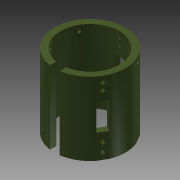
# Autodesk Inventor part: 知能ロボコン外筒改1.2
Saved by Autodesk Inventor 2013 (Build 170138000, 138)
## iProperties
Created: 2014-05-28
Part Number: 知能ロボコン外筒改1.2
Material: ABS プラスチック
Document SubType Name: Modeling
Designer: horumo136
Density: 1 g/cm^3
Author: horumo136
Autodesk Inventor part; units mm, degrees
sketch "スケッチ1" plane through (0, 0, 0) normal (0, 0, 1) x (1, 0, 0)
  circle A0 centre (0, 0) radius 13
  line L0 (0, 13) -> (0, 33)
  circle A1 centre (0, 0) radius 33
  circle A2 centre (0, 0) radius 40
  dimension "d0" = 26
  dimension "d2" = 20
  dimension "d3" = 80
  constraints: 3 coincident, 2 end point, 2 vertical alignment, 1 centre point, 1 vertical, 4 other
  measures "d2" distance of L0.start L0.end
  measures "d3" diameter of A2
extrude "押し出し1" add sketch "スケッチ1" along normal blind 145 contours A2
sketch "スケッチ2" plane through (0, 0, 0) normal (0, 0, -1) x (-1, 0, 0)
  circle A0 centre (0, 0) radius 33 projected
  circle A1 centre (0, 0) radius 40 projected
  line L0 (5.4, 32.5552) -> (-5.4, 32.5552)
  line L1 (0, 0) -> (-10.5703, 0)
  arc A2 (5.4, 32.5552) -> (-5.4, 32.5552) centre (0, 0) ccw
  line L2 (-5.4, 32.5552) -> (5.4, 32.5552)
  line L3 (5.4, 32.5552) -> (5.4, 32.5552)
  line L4 (5.4, 32.5552) -> (-5.4, 32.5552)
  line L5 (-5.4, 32.5552) -> (-5.4, 32.5552)
  line L6 (-5.4, 32.5552) -> (5.4, 32.5552)
  line L7 (5.4, 32.5552) -> (5.4, 33)
  line L8 (5.4, 33) -> (-5.4, 33)
  line L9 (-5.4, 33) -> (-5.4, 32.5552)
  line L10 (-30.8936, -11.6011) -> (-25.4936, -20.9541)
  line L11 (-30.8936, -11.6011) -> (-31.2788, -11.8235)
  line L12 (-31.2788, -11.8235) -> (-25.8788, -21.1765)
  line L13 (-25.8788, -21.1765) -> (-25.4936, -20.9541)
  line L14 (25.4936, -20.9541) -> (30.8936, -11.6011)
  line L15 (25.4936, -20.9541) -> (25.8788, -21.1765)
  line L16 (25.8788, -21.1765) -> (31.2788, -11.8235)
  line L17 (31.2788, -11.8235) -> (30.8936, -11.6011)
  line L18 (-30.8936, -11.6011) -> (-31.2788, -11.8235)
  line L19 (-31.2788, -11.8235) -> (-25.8788, -21.1765)
  line L20 (-25.8788, -21.1765) -> (-25.4936, -20.9541)
  line L21 (-25.4936, -20.9541) -> (-30.8936, -11.6011)
  line L22 (25.4936, -20.9541) -> (25.8788, -21.1765)
  line L23 (25.8788, -21.1765) -> (31.2788, -11.8235)
  line L24 (31.2788, -11.8235) -> (30.8936, -11.6011)
  line L25 (30.8936, -11.6011) -> (25.4936, -20.9541)
  dimension "d6" = 10.8
  dimension "d8" = 10.8
  dimension "d13" = 360
  constraints: 52 end point, 8 parallel, 6 perpendicular, 5 point on circle, 3 horizontal, 1 centre point, 1 collinear, 1 concentric, 31 other
  measures "d6" distance of L0.start L0.end
  measures "d8" distance of L4.end L3.end
extrude "押し出し2" cut sketch "スケッチ2" against normal blind 145 contours L0 A0 | A0 L8 L7 | L17 L16 A0 | A0 L14 | A0 L9 L8 | L16 L15 A0 | L10 A0 | A0 L12 L11 | L13 L12 A0
sketch "スケッチ3" plane through (-5.4, 33, 0) normal (0, -1, 0) x (1, 0, 0)
  line L0 (10.8, 0) -> (10.8, 145) projected
  line L1 (5.4, 0) -> (5.4, 19.5)
  line L2 (5.4, 19.5) -> (5.4, 24.2)
  line L3 (5.4, 24.2) -> (5.4, 74.8)
  circle A0 centre (5.4, 24.2) radius 1.5
  circle A1 centre (5.4, 74.8) radius 1.5
  line L4 (5.4, 74.8) -> (5.4, 79.9)
  line L5 (5.4, 79.9) -> (5.4, 84.6)
  circle A2 centre (5.4, 84.6) radius 1.5
  line L6 (5.4, 84.6) -> (5.4, 135.2)
  circle A3 centre (5.4, 135.2) radius 1.5
  dimension "d15" = 19.5
  dimension "d16" = 4.7
  dimension "d17" = 50.6
  dimension "d18" = 3
  dimension "d19" = 3
  dimension "d20" = 5.1
  dimension "d21" = 4.7
  dimension "d22" = 3
  dimension "d23" = 50.6
  dimension "d24" = 3
  constraints: 12 end point, 5 collinear, 4 centre point, 4 coincident, 1 parallel
  measures "d15" distance of L1.start L1.end
  measures "d16" distance of L1.end L2.end
  measures "d17" distance of L2.end L3.end
  measures "d18" diameter of A0
  measures "d19" diameter of A1
  measures "d20" distance of L4.start L4.end
  measures "d21" distance of L4.end L5.end
  measures "d22" diameter of A2
  measures "d23" distance of L6.start L6.end
  measures "d24" diameter of A3
hole "穴1" at (0, 33, 24.2) at (0, 33, 74.8) at (0, 33, 84.6) at (0, 33, 135.2) direction (0, 1, 0) diameter 3 depth 8 tip angle 118
pattern_circular "円形状パターン1" count 3 over 360 about axis through (0, 0, 0) along (0, 0, 1) of "穴1"
sketch "スケッチ4" plane through (0, 0, 0) normal (0, 0, -1) x (-1, 0, 0)
  circle A0 centre (0, 0) radius 40 projected
  line L0 (30.8936, -11.6011) -> (31.2788, -11.8235) projected
  line L1 (31.2788, -11.8235) -> (25.8788, -21.1765) projected
  line L2 (25.8788, -21.1765) -> (25.4936, -20.9541) projected
  arc A1 (-25.4936, -20.9541) -> (25.4936, -20.9541) centre (0, 0) ccw projected
  line L3 (-25.4936, -20.9541) -> (-25.8788, -21.1765) projected
  line L4 (-25.8788, -21.1765) -> (-31.2788, -11.8235) projected
  line L5 (-31.2788, -11.8235) -> (-30.8936, -11.6011) projected
  arc A2 (-5.4, 32.5552) -> (-30.8936, -11.6011) centre (0, 0) ccw projected
  line L6 (-5.4, 32.5552) -> (-5.4, 33) projected
  line L7 (-5.4, 33) -> (5.4, 33) projected
  line L8 (5.4, 33) -> (5.4, 32.5552) projected
  arc A3 (30.8936, -11.6011) -> (5.4, 32.5552) centre (0, 0) ccw projected
  point P0 (0, 40)
  point P1 (-34.641, 20)
  point P2 (-34.641, -20)
  point P3 (0, -40)
  point P4 (34.641, -20)
  point P5 (34.641, 20)
  dimension "d37" = 360
  constraints: 1 coincident, 1 vertical alignment, 8 other
ref_plane "作業平面1" through (-34.641, 20, 0) normal (-0.8660254, 0.5, 0) x (-0.5, -0.8660254, 0)
ref_plane "作業平面3" through (0, -40, 0) normal (0, -1, 0) x (1, 0, 0)
ref_plane "作業平面7" through (34.641, 20, 0) normal (0.8660254, 0.5, 0) x (-0.5, 0.8660254, 0)
sketch "スケッチ5" plane through (-34.641, 20, 0) normal (-0.8660254, 0.5, 0) x (-0.5, -0.8660254, 0)
  line L0 (0, 0) -> (0, 24.2)
  line L1 (0, 24.2) -> (0, 74.8)
  line L2 (0, 74.8) -> (0, 79.9)
  line L3 (0, 79.9) -> (0, 84.6)
  line L4 (0, 84.6) -> (0, 135.2)
  line L5 (-4, 139.2) -> (4, 139.2)
  line L6 (4, 139.2) -> (4, 131.2)
  line L7 (4, 131.2) -> (-4, 131.2)
  line L8 (-4, 131.2) -> (-4, 139.2)
  line L9 (-4, 139.2) -> (4, 131.2) construction
  line L10 (4, 139.2) -> (-4, 131.2) construction
  line L11 (-4, 89.6) -> (4, 89.6)
  line L12 (4, 89.6) -> (4, 79.6)
  line L13 (4, 79.6) -> (-4, 79.6)
  line L14 (-4, 79.6) -> (-4, 89.6)
  line L15 (-4, 89.6) -> (4, 79.6) construction
  line L16 (4, 89.6) -> (-4, 79.6) construction
  line L17 (-4, 79.8) -> (4, 79.8)
  line L18 (4, 79.8) -> (4, 69.8)
  line L19 (4, 69.8) -> (-4, 69.8)
  line L20 (-4, 69.8) -> (-4, 79.8)
  line L21 (-4, 79.8) -> (4, 69.8) construction
  line L22 (4, 79.8) -> (-4, 69.8) construction
  line L23 (-4, 28.2) -> (4, 28.2)
  line L24 (4, 28.2) -> (4, 20.2)
  line L25 (4, 20.2) -> (-4, 20.2)
  line L26 (-4, 20.2) -> (-4, 28.2)
  line L27 (-4, 28.2) -> (4, 20.2) construction
  line L28 (4, 28.2) -> (-4, 20.2) construction
  dimension "d39" = 24.2
  dimension "d40" = 50.6
  dimension "d41" = 5.1
  dimension "d42" = 4.7
  dimension "d43" = 50.6
  dimension "d44" = 8
  dimension "d45" = 8
  dimension "d46" = 8
  dimension "d47" = 10
  dimension "d48" = 8
  dimension "d49" = 10
  dimension "d50" = 8
  dimension "d51" = 8
  constraints: 58 end point, 8 midpoint, 8 parallel, 4 horizontal, 4 perpendicular, 3 collinear, 1 point on line, 1 vertical
  measures "d39" distance of L0.start L0.end
  measures "d40" distance of L0.end L1.end
  measures "d41" distance of L1.end L2.end
  measures "d42" distance of L2.end L3.end
  measures "d43" distance of L3.end L4.end
  measures "d44" distance of L6.end L7.end
  measures "d45" distance of L5.end L6.end
  measures "d46" distance of L12.end L13.end
  measures "d47" distance of L11.end L12.end
  measures "d48" distance of L18.end L19.end
  measures "d49" distance of L17.end L18.end
  measures "d50" distance of L24.end L25.end
  measures "d51" distance of L23.end L24.end
extrude "押し出し3" [suppressed]
pattern_circular "円形状パターン2" [suppressed]
ref_plane "作業平面8" through (0, 40, 0) normal (0, 1, 0) x (-1, 0, 0)
sketch "スケッチ6" plane through (0, 40, 0) normal (0, 1, 0) x (-1, 0, 0)
  line L0 (0, 0) -> (0, 24.2)
  line L1 (0, 24.2) -> (0, 74.8)
  line L2 (0, 74.8) -> (0, 84.6)
  line L3 (0, 84.6) -> (0, 135.2)
  dimension "d57" = 24.2
  dimension "d58" = 50.6
  dimension "d59" = 9.8
  dimension "d60" = 50.6
  constraints: 8 end point, 4 coincident, 3 collinear, 1 vertical
  measures "d57" distance of L0.start L0.end
  measures "d58" distance of L0.end L1.end
  measures "d59" distance of L1.end L2.end
  measures "d60" distance of L2.end L3.end
hole "穴2" at (0, 40, 74.8) at (0, 40, 24.2) at (0, 40, 84.6) at (0, 40, 135.2) direction (0, -1, 0) diameter 3 depth 8 tip angle 118 counterbore diameter 4 counterbore depth 2
pattern_circular "円形状パターン3" count 3 over 360 about axis through (0, 0, 0) along (0, 0, 1) of "穴2"
sketch "スケッチ7" plane through (0, -40, 0) normal (0, -1, 0) x (1, 0, 0)
  line L0 (0, 0) -> (-5.5, 0)
  line L1 (-5.5, 0) -> (5.5, 0)
  line L2 (-5.5, 0) -> (5.5, 0)
  line L3 (5.5, 0) -> (5.5, 150)
  line L4 (5.5, 150) -> (-5.5, 150)
  line L5 (-5.5, 150) -> (-5.5, 0)
  line L6 (-5.5, 150) -> (5.5, 150)
  line L7 (5.5, 150) -> (5.5, 10)
  line L8 (5.5, 10) -> (-5.5, 10)
  line L9 (-5.5, 10) -> (-5.5, 150)
  dimension "d71" = 5.5
  dimension "d72" = 11
  dimension "d73" = 11
  dimension "d74" = 150
  dimension "d75" = 10
  constraints: 20 end point, 4 parallel, 3 horizontal, 2 perpendicular, 1 collinear, 1 point on line
  measures "d71" distance of L0.start L0.end
  measures "d72" distance of L0.end L1.end
  measures "d73" distance of L4.end L3.end
  measures "d74" distance of L3.end L2.end
  measures "d75" distance between parallel lines of L2 L8
extrude "押し出し4" cut sketch "スケッチ7" against normal blind 10 contours L5 L4 L3 L8
sketch "スケッチ8" plane through (0, 0, 0) normal (0, 0, -1) x (-1, 0, 0)
  circle A0 centre (0, 0) radius 40 projected
  line L0 (5.4, 33) -> (5.4, 32.5552) projected
  line L1 (-5.4, 39.6338) -> (5.4, 39.6338)
  arc A1 (5.4, 39.6338) -> (-5.4, 39.6338) centre (0, 0) ccw
  constraints: 4 point on circle, 2 end point, 1 centre point, 1 concentric, 1 perpendicular
extrude "押し出し5" cut sketch "スケッチ8" against normal blind 145 contours L1 A0 picked at (-0.6016, 39.7423)
sketch "スケッチ9" plane through (0, 0, 0) normal (0, 0, -1) x (-1, 0, 0)
  line L0 (30.8936, -11.6011) -> (31.2788, -11.8235) projected
  line L1 (31.2788, -11.8235) -> (25.8788, -21.1765) projected
  line L2 (25.8788, -21.1765) -> (25.4936, -20.9541) projected
  arc A0 (-25.4936, -20.9541) -> (25.4936, -20.9541) centre (0, 0) ccw projected
  line L3 (-25.4936, -20.9541) -> (-25.8788, -21.1765) projected
  line L4 (-25.8788, -21.1765) -> (-31.2788, -11.8235) projected
  line L5 (-31.2788, -11.8235) -> (-30.8936, -11.6011) projected
  arc A1 (-5.4, 32.5552) -> (-30.8936, -11.6011) centre (0, 0) ccw projected
  line L6 (-5.4, 32.5552) -> (-5.4, 33) projected
  line L7 (-5.4, 33) -> (5.4, 33) projected
  line L8 (5.4, 33) -> (5.4, 32.5552) projected
  arc A2 (30.8936, -11.6011) -> (5.4, 32.5552) centre (0, 0) ccw projected
  line L9 (-45, -40) -> (45, -40)
  line L10 (45, -40) -> (45, 40)
  line L11 (45, 40) -> (-45, 40)
  line L12 (-45, 40) -> (-45, -40)
  line L13 (-45, -40) -> (45, 40) construction
  line L14 (45, -40) -> (-45, 40) construction
  dimension "d80" = 90
  dimension "d81" = 80
  constraints: 12 end point, 2 midpoint, 2 parallel, 1 horizontal, 1 perpendicular
  measures "d80" distance of L11.end L10.end
  measures "d81" distance of L10.end L9.end
extrude "押し出し6" add sketch "スケッチ9" along normal blind 5
sketch "スケッチ10" plane through (0, 0, 145) normal (0, 0, 1) x (1, 0, 0)
  line L0 (5.4, 39.6338) -> (-5.4, 39.6338) projected
  arc A0 (-5.4, 39.6338) -> (-5.5, -39.6201) centre (0, 0) ccw projected
  line L1 (-5.5, -39.6201) -> (-5.5, -32.5384) projected
  arc A1 (-25.4936, -20.9541) -> (-5.5, -32.5384) centre (0, 0) ccw projected
  line L2 (-25.4936, -20.9541) -> (-25.8788, -21.1765) projected
  line L3 (-25.8788, -21.1765) -> (-31.2788, -11.8235) projected
  line L4 (-31.2788, -11.8235) -> (-30.8936, -11.6011) projected
  arc A2 (-5.4, 32.5552) -> (-30.8936, -11.6011) centre (0, 0) ccw projected
  line L5 (-5.4, 32.5552) -> (-5.4, 33) projected
  line L6 (-5.4, 33) -> (5.4, 33) projected
  line L7 (5.4, 33) -> (5.4, 32.5552) projected
  arc A3 (30.8936, -11.6011) -> (5.4, 32.5552) centre (0, 0) ccw projected
  line L8 (30.8936, -11.6011) -> (31.2788, -11.8235) projected
  line L9 (31.2788, -11.8235) -> (25.8788, -21.1765) projected
  line L10 (25.8788, -21.1765) -> (25.4936, -20.9541) projected
  arc A4 (5.5, -32.5384) -> (25.4936, -20.9541) centre (0, 0) ccw projected
  line L11 (5.5, -32.5384) -> (5.5, -39.6201) projected
  arc A5 (5.5, -39.6201) -> (5.4, 39.6338) centre (0, 0) ccw projected
  line L12 (-45, 40) -> (45, 40)
  line L13 (45, 40) -> (45, -40)
  line L14 (45, -40) -> (-45, -40)
  line L15 (-45, -40) -> (-45, 40)
  line L16 (-45, 40) -> (45, -40) construction
  line L17 (45, 40) -> (-45, -40) construction
  line L18 (-5.5, -32.5384) -> (-5.5, -40)
  line L19 (-5.5, -40) -> (-45, -40)
  line L20 (-45, -40) -> (-45, 40)
  line L21 (-45, 40) -> (45, 40)
  line L22 (45, 40) -> (45, -40)
  line L23 (45, -40) -> (5.5, -40)
  line L24 (5.5, -40) -> (5.5, -32.5384)
  arc A6 (5.5, -32.5384) -> (-5.5, -32.5384) centre (0, 0) ccw
  circle A7 centre (0, 0) radius 33
  line L25 (-5.5, -40) -> (5.5, -40)
  dimension "d84" = 90
  dimension "d85" = 80
  constraints: 28 end point, 4 collinear, 3 parallel, 2 concentric, 2 midpoint, 2 perpendicular, 2 point on circle, 2 point on line, 1 centre point, 1 coincident, 1 horizontal, 3 other
  measures "d84" distance of L13.end L14.end
  measures "d85" distance of L12.end L13.end
extrude "押し出し7" add sketch "スケッチ10" along normal blind 5 contours A5 L11 A4 L10 L9 L8 A3 L7 L6 L5 A2 L4 L3 L2 A1 L1 A0 L0 | L0 A0 L18 L14 L15 L12 L13 L24 A5 | L24 L14 L18 L1 A7 L11
sketch "スケッチ11" plane through (-5.4, 39.6338, 0) normal (0, 1, 0) x (1, 0, 0)
  circle A0 centre (5.4, -84.6) radius 2 projected
  circle A1 centre (5.4, -74.8) radius 2 projected
  circle A2 centre (5.4, -24.2) radius 2 projected
  circle A3 centre (5.4, -135.2) radius 2 projected
  line L0 (0, 0) -> (10.8, 0) projected
  line L1 (0, -145) -> (0, 0) projected
  line L2 (10.8, -145) -> (0, -145) projected
  line L3 (10.8, 0) -> (10.8, -145) projected
  line L4 (5.4, 0) -> (5.4, -145)
  line L5 (5.4, 0) -> (5.4, -72.5)
  dimension "d88" = 72.5
  constraints: 4 end point, 2 midpoint
  measures "d88" distance of L4.start L5.end
ref_plane "作業平面9" through (0, 39.6338, 72.5) normal (0, 0, -1) x (-1, 0, 0)
sketch "スケッチ12" plane through (0, 39.6338, 72.5) normal (0, 0, -1) x (-1, 0, 0)
  line L0 (-45, -79.6338) -> (45, -79.6338)
  line L1 (45, -79.6338) -> (45, 0.3662)
  line L2 (45, 0.3662) -> (-45, 0.3662)
  line L3 (-45, 0.3662) -> (-45, -79.6338)
  line L4 (-45, -79.6338) -> (45, 0.3662) construction
  line L5 (45, -79.6338) -> (-45, 0.3662) construction
  point P0 (0, -39.6338)
  dimension "d89" = 90
  dimension "d90" = 80
  constraints: 12 end point, 2 midpoint, 2 parallel, 1 horizontal, 1 perpendicular
  measures "d89" distance of L2.end L1.end
  measures "d90" distance of L1.end L0.end
extrude "押し出し8" cut sketch "スケッチ12" along normal blind 80
sketch "スケッチ13" plane through (0, 39.6338, 72.5) normal (0, 0, -1) x (-1, 0, 0)
  line L0 (-31.2788, -51.4573) -> (-25.8788, -60.8104) projected
  line L1 (-30.8936, -51.2349) -> (-31.2788, -51.4573) projected
  arc A0 (-5.4, -7.0786) -> (-30.8936, -51.2349) centre (0, -39.6338) ccw projected
  line L2 (-5.4, -6.6338) -> (-5.4, -7.0786) projected
  line L3 (5.4, -6.6338) -> (-5.4, -6.6338) projected
  line L4 (5.4, -7.0786) -> (5.4, -6.6338) projected
  arc A1 (30.8936, -51.2349) -> (5.4, -7.0786) centre (0, -39.6338) ccw projected
  line L5 (31.2788, -51.4573) -> (30.8936, -51.2349) projected
  line L6 (25.8788, -60.8104) -> (31.2788, -51.4573) projected
  line L7 (25.4936, -60.588) -> (25.8788, -60.8104) projected
  arc A2 (5.5, -72.1723) -> (25.4936, -60.588) centre (0, -39.6338) ccw projected
  line L8 (5.5, -79.2539) -> (5.5, -72.1723) projected
  arc A3 (5.5, -79.2539) -> (5.4, 0) centre (0, -39.6338) ccw projected
  line L9 (-5.4, 0) -> (5.4, 0) projected
  arc A4 (-5.4, 0) -> (-5.5, -79.2539) centre (0, -39.6338) ccw projected
  line L10 (-5.5, -72.1723) -> (-5.5, -79.2539) projected
  arc A5 (-25.4936, -60.588) -> (-5.5, -72.1723) centre (0, -39.6338) ccw projected
  line L11 (-25.8788, -60.8104) -> (-25.4936, -60.588) projected
extrude "押し出し9" add sketch "スケッチ13" along normal blind 5
sketch "スケッチ14" plane through (-5.4, 33, 150) normal (0, -1, 0) x (1, 0, 0)
  line L0 (10.8, -82.5) -> (10.8, 0) projected
  circle A0 centre (5.4, -14.8) radius 1.5 projected
  circle A1 centre (5.4, -65.4) radius 1.5 projected
  line L1 (5.4, -14.8) -> (5.4, -65.4)
  line L2 (0, -25.1) -> (10.8, -25.1)
  line L3 (10.8, -25.1) -> (10.8, -55.1)
  line L4 (10.8, -55.1) -> (0, -55.1)
  line L5 (0, -55.1) -> (0, -25.1)
  line L6 (0, -25.1) -> (10.8, -55.1) construction
  line L7 (10.8, -25.1) -> (0, -55.1) construction
  point P0 (5.4, -150)
  point P1 (5.4, -40.1)
  dimension "d95" = 30
  constraints: 14 end point, 3 midpoint, 3 parallel, 1 horizontal, 1 perpendicular, 1 point on line
  measures "d95" distance of L2.end L3.end
extrude "押し出し10" cut sketch "スケッチ14" against normal blind 10 contours L4 L1 L2 L0 | L4 L5 L2 L1
sketch "スケッチ15" plane through (25.8788, -21.1765, 67.5) normal (-0.8660254, 0.5, 0) x (0, 0, 1)
  line L0 (0, 0) -> (82.5, 0) projected
  line L1 (0, 0) -> (0, 10.8) projected
  circle A0 centre (17.1, 5.4) radius 1.5 projected
  circle A1 centre (67.7, 5.4) radius 1.5 projected
  line L2 (67.7, 5.4) -> (17.1, 5.4)
  line L3 (27.4, 10.8) -> (57.4, 10.8)
  line L4 (57.4, 10.8) -> (57.4, 0)
  line L5 (57.4, 0) -> (27.4, 0)
  line L6 (27.4, 0) -> (27.4, 10.8)
  line L7 (27.4, 10.8) -> (57.4, 0) construction
  line L8 (57.4, 10.8) -> (27.4, 0) construction
  point P0 (-67.5, 5.4)
  point P1 (42.4, 5.4)
  dimension "d98" = 30
  constraints: 14 end point, 3 midpoint, 2 parallel, 2 perpendicular, 1 horizontal, 1 point on line
  measures "d98" distance of L4.end L5.end
extrude "押し出し11" cut sketch "スケッチ15" against normal blind 10 contours L6 L2 L4 L0 | L6 L3 L4 L2
sketch "スケッチ16" plane through (-31.2788, -11.8235, 150) normal (0.8660254, 0.5, 0) x (0, 0, -1)
  line L0 (0, -10.8) -> (82.5, -10.8) projected
  line L1 (82.5, 0) -> (82.5, -10.8) projected
  circle A0 centre (14.8, -5.4) radius 1.5 projected
  circle A1 centre (65.4, -5.4) radius 1.5 projected
  line L2 (14.8, -5.4) -> (65.4, -5.4)
  line L3 (25.1, 0) -> (55.1, 0)
  line L4 (55.1, 0) -> (55.1, -10.8)
  line L5 (55.1, -10.8) -> (25.1, -10.8)
  line L6 (25.1, -10.8) -> (25.1, 0)
  line L7 (25.1, 0) -> (55.1, -10.8) construction
  line L8 (55.1, 0) -> (25.1, -10.8) construction
  point P0 (150, -5.4)
  point P1 (40.1, -5.4)
  dimension "d101" = 30
  constraints: 14 end point, 3 midpoint, 2 parallel, 2 perpendicular, 1 horizontal, 1 point on line
  measures "d101" distance of L4.end L5.end
extrude "押し出し12" cut sketch "スケッチ16" against normal blind 10 contours L6 L2 L4 L0 | L6 L3 L4 L2
sketch "スケッチ17" plane through (0, 0, 150) normal (0, 0, 1) x (1, 0, 0)
  line L0 (-45, 40) -> (-35, 40)
  line L1 (-35, 40) -> (-35, 30)
  line L2 (-35, 30) -> (-45, 30)
  line L3 (-45, 30) -> (-45, 40)
  line L4 (45, 40) -> (35, 40)
  line L5 (35, 40) -> (35, 30)
  line L6 (35, 30) -> (45, 30)
  line L7 (45, 30) -> (45, 40)
  line L8 (45, -40) -> (35, -40)
  line L9 (35, -40) -> (35, -30)
  line L10 (35, -30) -> (45, -30)
  line L11 (45, -30) -> (45, -40)
  line L12 (-45, -40) -> (-35, -40)
  line L13 (-35, -40) -> (-35, -30)
  line L14 (-35, -30) -> (-45, -30)
  line L15 (-45, -30) -> (-45, -40)
  dimension "d104" = 10
  dimension "d105" = 10
  dimension "d106" = 10
  dimension "d107" = 10
  dimension "d108" = 10
  dimension "d109" = 10
  dimension "d110" = 10
  dimension "d111" = 10
  constraints: 32 end point, 8 parallel, 5 coincident, 4 horizontal, 4 perpendicular
  measures "d104" distance of L1.end L2.end
  measures "d105" distance of L0.end L1.end
  measures "d106" distance of L6.end L5.end
  measures "d107" distance of L5.end L4.end
  measures "d108" distance of L9.end L10.end
  measures "d109" distance of L8.end L9.end
  measures "d110" distance of L14.end L13.end
  measures "d111" distance of L13.end L12.end
hole "穴3" at (-35, -30, 150) at (-35, 30, 150) at (35, -30, 150) at (35, 30, 150) direction (0, 0, -1) diameter 3 depth 8 tip angle 118
sketch "スケッチ18" plane through (0, 0, 150) normal (0, 0, 1) x (1, 0, 0)
  circle A0 centre (35, -30) radius 1.5 projected
  circle A1 centre (-35, -30) radius 1.5 projected
  circle A2 centre (-35, 30) radius 1.5 projected
  circle A3 centre (35, 30) radius 1.5 projected
  line L0 (-45, -40) -> (45, -40) projected
  line L1 (45, -40) -> (45, 40) projected
  line L2 (45, 40) -> (-45, 40) projected
  line L3 (-45, 40) -> (-45, -40) projected
  arc A4 (-5.4, 32.5552) -> (-30.8936, -11.6011) centre (0, 0) ccw projected
  circle A5 centre (0, 0) radius 40
  dimension "d119" = 80
  constraints: 1 centre point, 1 coincident
  measures "d119" diameter of A5
extrude "押し出し13" cut sketch "スケッチ18" against normal blind 10 contours L3 L2 A5 L0 | A5 L2 L1 L0
sketch "スケッチ19" plane through (0, 0, 145) normal (0, 0, -1) x (-1, 0, 0)
  arc A0 (-5.5, -39.6201) -> (5.5, -39.6201) centre (0, 0) ccw projected
  line L0 (5.5, -39.6201) -> (5.5, -32.5384) projected
  arc A1 (-5.5, -32.5384) -> (5.5, -32.5384) centre (0, 0) ccw projected
  line L1 (-5.5, -32.5384) -> (-5.5, -39.6201) projected
extrude "押し出し14" cut sketch "スケッチ19" against normal blind 10
sketch "スケッチ20" plane through (0, 0, 145) normal (0, 0, -1) x (-1, 0, 0)
  arc A0 (5.4, 39.6338) -> (-5.4, 39.6338) centre (0, 0) ccw projected
  line L0 (-5.4, 39.6338) -> (5.4, 39.6338) projected
extrude "押し出し15" cut sketch "スケッチ20" against normal blind 10
sketch "スケッチ21" plane through (-5.4, 39.6338, 150) normal (0, 1, 0) x (1, 0, 0)
  line L0 (10.8, 25.1) -> (10.8, 0) projected
  circle A0 centre (5.4, 14.8) radius 2 projected
  line L1 (5.4, 14.8) -> (5.4, 6.8)
  point P0 (5.4, 150)
  dimension "d126" = 8
  constraints: 2 end point, 1 coincident, 1 parallel
  measures "d126" distance of L1.start L1.end
hole "穴4" at (0, 39.6338, 143.2) direction (0, -1, 0) diameter 3 depth 8 tip angle 118 counterbore diameter 4 counterbore depth 2
pattern_circular "円形状パターン4" count 6 over 360 about axis through (0, 0, 0) along (0, 0, 1) of "穴4"
pattern_circular "円形状パターン5" count 6 over 360 about axis through (0, 0, 0) along (0, 0, 1) of "押し出し5"
